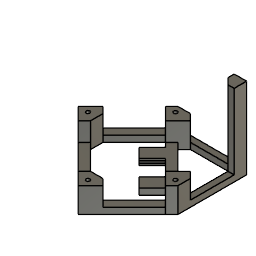
台1 v10 (Autodesk Fusion 360 design; units mm, degrees)
Autodesk Fusion 360 part; units mm, degrees
sketch "スケッチ1" plane through (0, 0, 0) normal (0, 0, 1) x (1, 0, 0)
  line L0 (0, 0) -> (-55, 0)
  line L1 (0, 0) -> (0, -5)
  line L2 (-10, -5) -> (-50, -5)
  line L3 (0, 0) -> (0, -55)
  line L4 (-5, -50) -> (-5, -10)
  line L5 (-5, -10) -> (-10, -5)
  line L6 (-5, -50) -> (-50, -5)
  line L7 (-5, -60) -> (-60, -5)
  line L8 (-60, -5) -> (-55, 0)
  line L9 (0, -55) -> (-5, -60)
  constraint coincident L0.start L1.start
  constraint horizontal L0
  constraint perpendicular L0 L1
  constraint perpendicular L1 L2
  constraint perpendicular L0 L3
  constraint perpendicular L2 L4
  constraint parallel L6 L7
  constraint perpendicular L6 L8
  constraint perpendicular L7 L9
extrude "押し出し1" add sketch "スケッチ1" along normal blind 5
sketch "スケッチ2" plane through (0, 0, 0) normal (0, 0, 1) x (1, 0, 0)
  line L0 (0, 0, 5) -> (-55, 0, 5)
  line L1 (-10, -5, 5) -> (-10, 0, 5)
  line L2 (-10, -5, 5) -> (-5, -10, 5)
  line L3 (0, -55, 5) -> (0, 0, 5)
  line L4 (-5, -10, 5) -> (0, -10, 5)
  line L5 (-60, -5, 5) -> (-5, -60, 5)
  line L6 (-5, -60, 5) -> (0, -55, 5)
  line L7 (-55, 0, 5) -> (-60, -5, 5)
  line L8 (-10, -55, 5) -> (-15, -50, 5)
  line L9 (-5, -10, 5) -> (-5, -50, 5)
  line L10 (0, -45, 5) -> (-5, -40, 5)
  line L11 (-15, -50, 5) -> (-5, -40, 5)
  line L12 (-50, -5, 5) -> (-10, -5, 5)
  line L13 (-50, -15, 5) -> (-40, -5, 5)
  line L14 (-45, 0, 5) -> (-40, -5, 5)
  line L15 (-55, -10, 5) -> (-50, -15, 5)
  point P0 (-10, -5)
  point P1 (-10, -5)
  point P2 (-5, -10)
  point P3 (-5, -50)
  point P4 (-50, -5)
  constraint coincident P0 P1
  constraint coincident P1 P0
extrude "押し出し2" add sketch "スケッチ2" along normal blind 50 contours L0 L1 L2 L3 L4 | L0 L5 L7 L13 L14 L15 | L3 L5 L6 L8 L10 L11 in plane through (0, 0, 5) normal (0, 0, 1)
sketch "スケッチ3" plane through (0, 0, 0) normal (0, 0, 1) x (1, 0, 0)
extrude "押し出し3" cut 2 faces at (-50, -5, 55) (-5, -50, 55) along direction (0, 0, -1) blind 30
sketch "スケッチ4" plane through (0, 0, 0) normal (0, 0, 1) x (1, 0, 0)
  line L0 (-60, -5) -> (-95, -40)
  line L1 (-95, -40) -> (-40, -95)
  line L2 (-40, -95) -> (-5, -60)
  line L3 (-5, -60) -> (-60, -5)
  line L4 (-55, -10) -> (-80, -35)
  line L5 (-80, -45) -> (-45, -80)
  line L6 (-35, -80) -> (-10, -55)
  line L7 (-35, -80) -> (-45, -80)
  line L8 (-80, -35) -> (-80, -45)
  point P0 (-5, -60)
  constraint perpendicular L0 L1
  constraint coincident P0 L2.end
  constraint coincident L3 L4.start
  constraint perpendicular L3 L4
  constraint perpendicular L4 L5
  constraint coincident L3 L6.end
  constraint perpendicular L3 L6
  constraint horizontal L7
  constraint perpendicular L7 L8
extrude "押し出し4" add sketch "スケッチ4" along normal blind 5 contours L0 L1 L2 L3 L4 L5 L6 L7 L8
sketch "スケッチ5" plane through (0, 0, 5) normal (0, 0, 1) x (-1, 0, 0)
  line L0 (55, 10) -> (60, 5)
  line L1 (60, 5) -> (95, 40)
  line L2 (95, 40) -> (40, 95)
  line L3 (40, 95) -> (5, 60)
  line L4 (10, 55) -> (35, 80)
  line L5 (35, 80) -> (45, 80)
  line L6 (45, 80) -> (80, 45)
  line L7 (80, 45) -> (80, 35)
  line L8 (80, 35) -> (55, 10)
  line L9 (80, 35) -> (85, 30)
  line L10 (80, 45) -> (85, 50)
  line L11 (45, 80) -> (50, 85)
  line L12 (35, 80) -> (30, 85)
  line L13 (5, 60) -> (10, 55)
  constraint coincident L7.end L8.start
  constraint coincident L1 L9.end
  constraint perpendicular L1 L9
  constraint coincident L6.end L7.start
  constraint coincident L2 L10.end
  constraint perpendicular L2 L10
  constraint coincident L5.end L6.start
  constraint coincident L2 L11.end
  constraint perpendicular L2 L11
  constraint coincident L4.end L5.start
  constraint coincident L3 L12.end
  constraint perpendicular L3 L12
extrude "押し出し5" add sketch "スケッチ5" along normal blind 20 contours L1 L2 L7 L9 L10 | L2 L3 L5 L11 L12
extrude "押し出し6" cut 4 faces at (-50, -5, 25) (-85, -40, 25) (-40, -85, 25) (-5, -50, 25) along direction (0, 0, -1) blind 5
extrude "押し出し7" add 2 faces at (-6.6667, -45, 5) (-45, -6.6667, 5) along direction (0, 0, -1) blind 5
sketch "スケッチ6" plane through (0, 0, 20) normal (0, 0, 1) x (-1, 0, 0)
  line L0 (45, 80) -> (50, 85)
  line L1 (50, 85) -> (40, 95)
  line L2 (40, 95) -> (30, 85)
  line L3 (30, 85) -> (35, 80)
  line L4 (35, 80) -> (45, 80)
  circle A0 centre (40, 87) radius 1.5
  circle A1 centre (5, 52) radius 1.5
  circle A2 centre (87, 40) radius 1.5
  circle A3 centre (52, 5) radius 1.5
extrude "押し出し8" cut sketch "スケッチ6" against normal blind 10 contours A0 | A1 | A2 | A3
sketch "スケッチ7" plane through (0, 0, 10) normal (0, 0, 1) x (-1, 0, 0)
  circle A0 centre (40, 87) radius 1.5
  circle A1 centre (40, 87) radius 2.5
  circle A2 centre (87, 40) radius 2.5
  circle A3 centre (87, 40) radius 1.5
  circle A4 centre (5, 52) radius 2.5
  circle A5 centre (5, 52) radius 1.5
  circle A6 centre (52, 5) radius 2.5
  circle A7 centre (52, 5) radius 1.5
  constraint concentric A0 A1
  constraint concentric A2 A3
  constraint concentric A4 A5
  constraint concentric A6 A7
extrude "押し出し9" cut sketch "スケッチ7" against normal blind 10 contours A0 | A1 | A2 | A3 | A4 | A5 | A6 | A7
extrude "押し出し10" cut 4 faces at (-38.0024, -87.8241, 10) (-2.8482, -51.8013, 10) (-54.1518, -4.8013, 10) (-85.2875, -41.3179, 10) along direction (0, 0, 1) blind 5
extrude "押し出し11" add 1 faces at (-5, -5, 55) along direction (0, 0, 1) blind 30
sketch "スケッチ8" plane through (-7.5, -7.5, 0) normal (-0.707107, -0.707107, 0) x (0.707107, -0.707107, 0)
  line L0 (-3.5355, 0) -> (3.5355, 0)
  line L1 (3.5355, 0) -> (3.5355, 5)
  line L2 (3.5355, 5) -> (3.5355, 85)
  line L3 (3.5355, 85) -> (-3.5355, 85)
  line L4 (-3.5355, 85) -> (-3.5355, 5)
  line L5 (-3.5355, 5) -> (-3.5355, 0)
  line L6 (0, 35) -> (0, 25)
  line L7 (-1.5, 35) -> (-1.5, 25)
  arc A0 (-1.5, 25) -> (1.5, 25) centre (0, 25) ccw
  line L8 (1.5, 25) -> (1.5, 35)
  arc A1 (1.5, 35) -> (-1.5, 35) centre (0, 35) ccw
  line L9 (0, 35) -> (0, 25) construction
  constraint perpendicular L0 L6
  constraint tangent L7 A0
  constraint tangent A0 L8
  constraint parallel L7 L8
  constraint tangent L8 A1
  constraint tangent L7 A1
  constraint coincident L6.end A0.centre
  constraint parallel L6 L9
  constraint coincident L6.start A1.centre
extrude "押し出し12" cut sketch "スケッチ8" against normal blind 4 contours L7 A0 L8 A1
sketch "スケッチ9" plane through (-32.5, -32.5, 0) normal (-0.707107, -0.707107, 0) x (0.707107, -0.707107, 0)
  line L0 (-24.7487, 20) -> (-38.8909, 20)
  line L1 (-38.8909, 20) -> (-38.8909, 5)
  line L2 (-38.8909, 5) -> (-31.8198, 5)
  line L3 (-31.8198, 5) -> (-31.8198, 0)
  line L4 (-31.8198, 0) -> (31.8198, 0)
  line L5 (31.8198, 0) -> (31.8198, 5)
  line L6 (31.8198, 5) -> (38.8909, 5)
  line L7 (38.8909, 5) -> (38.8909, 20)
  line L8 (38.8909, 20) -> (24.7487, 20)
  line L9 (24.7487, 20) -> (24.7487, 5)
  line L10 (24.7487, 5) -> (-24.7487, 5)
  line L11 (-24.7487, 5) -> (-24.7487, 20)
  line L12 (-9, 5) -> (-20, 5)
  line L13 (-20, 5) -> (-20, 0)
  line L14 (-20, 0) -> (-9, 0)
  line L15 (-9, 0) -> (-9, 5)
  line L16 (9, 5) -> (20, 5)
  line L17 (20, 5) -> (20, 0)
  line L18 (20, 0) -> (9, 0)
  line L19 (9, 0) -> (9, 5)
  constraint horizontal L12
  constraint vertical L13
  constraint horizontal L14
  constraint vertical L15
  constraint coincident L4 L13.end
  constraint coincident L10 L12.start
  constraint horizontal L16
  constraint vertical L17
  constraint horizontal L18
  constraint vertical L19
  constraint coincident L4 L17.end
  constraint coincident L10 L16.start
extrude "押し出し13" add sketch "スケッチ9" along normal blind 20 contours L4 L10 L12 L13 L14 L15 | L4 L10 L16 L17 L18 L19
sketch "スケッチ10" plane through (-46.6421, -46.6421, 0) normal (-0.707107, -0.707107, 0) x (0.707107, -0.707107, 0)
  line L0 (-9, 0) -> (-9, 5)
  line L1 (-9, 5) -> (-20, 5)
  line L2 (-20, 5) -> (-20, 0)
  line L3 (-20, 0) -> (-9, 0)
  line L4 (-9.5, 2.5) -> (9.5, 2.5)
  line L5 (-9.5, 1.5) -> (9.5, 1.5)
  arc A0 (9.5, 1.5) -> (9.5, 3.5) centre (9.5, 2.5) ccw
  line L6 (9.5, 3.5) -> (-9.5, 3.5)
  arc A1 (-9.5, 3.5) -> (-9.5, 1.5) centre (-9.5, 2.5) ccw
  line L7 (-9.5, 2.5) -> (9.5, 2.5) construction
  constraint perpendicular L0 L4
  constraint tangent L5 A0
  constraint tangent A0 L6
  constraint parallel L5 L6
  constraint tangent L6 A1
  constraint tangent L5 A1
  constraint coincident L4.end A0.centre
  constraint perpendicular L0 L7
  constraint coincident L4.start A1.centre
extrude "押し出し14" cut sketch "スケッチ10" against normal blind 20 contours L0 L5 L6 A1 | L0 L5 A0 L6
extrude "押し出し15" cut 2 faces at (-58.5444, -34.7398, 2.5249) (-34.7398, -58.5444, 2.4751) along direction (0.707107, 0.707107, 0) blind 5
sketch "スケッチ11" plane through (0, 0, 0) normal (0, 0, -1) x (1, 0, 0)
  line L0 (-49.4706, 36.7426) -> (-57.2487, 28.9645)
  line L1 (-57.2487, 28.9645) -> (-46.6421, 18.3579)
  line L2 (-46.6421, 18.3579) -> (-55, 10)
  line L3 (-55, 10) -> (-80, 35)
  line L4 (-80, 35) -> (-80, 45)
  line L5 (-80, 45) -> (-45, 80)
  line L6 (-45, 80) -> (-35, 80)
  line L7 (-35, 80) -> (-10, 55)
  line L8 (-10, 55) -> (-18.3579, 46.6421)
  line L9 (-18.3579, 46.6421) -> (-28.9645, 57.2487)
  line L10 (-28.9645, 57.2487) -> (-36.7426, 49.4706)
  line L11 (-36.7426, 49.4706) -> (-26.136, 38.864)
  line L12 (-26.136, 38.864) -> (-38.864, 26.136)
  line L13 (-38.864, 26.136) -> (-49.4706, 36.7426)
  line L14 (-5, 60) -> (-40, 95)
  line L15 (-40, 95) -> (-95, 40)
  line L16 (-95, 40) -> (-55, 0)
  line L17 (-55, 0) -> (0, 0)
  line L18 (0, 0) -> (0, 55)
  line L19 (0, 55) -> (-5, 60)
  line L20 (-5, 10) -> (-10, 5)
  line L21 (-10, 5) -> (-40, 5)
  line L22 (-40, 5) -> (-45, 10)
  line L23 (-45, 10) -> (-10, 45)
  line L24 (-10, 45) -> (-5, 40)
  line L25 (-5, 40) -> (-5, 10)
  circle A0 centre (-40, 87) radius 2.5
  circle A1 centre (-87, 40) radius 2.5
  circle A2 centre (-5, 52) radius 2.5
  circle A3 centre (-52, 5) radius 2.5
extrude "押し出し16" cut 1 faces at (-5, -5, 85) along direction (0, 0, -1) blind 20
sketch "スケッチ12" plane through (0, 0, 0) normal (0, 0, -1) x (1, 0, 0)
  line L0 (-49.4706, 36.7426) -> (-57.2487, 28.9645)
  line L1 (-57.2487, 28.9645) -> (-46.6421, 18.3579)
  line L2 (-46.6421, 18.3579) -> (-55, 10)
  line L3 (-55, 10) -> (-80, 35)
  line L4 (-80, 35) -> (-80, 45)
  line L5 (-80, 45) -> (-45, 80)
  line L6 (-45, 80) -> (-35, 80)
  line L7 (-35, 80) -> (-10, 55)
  line L8 (-10, 55) -> (-18.3579, 46.6421)
  line L9 (-18.3579, 46.6421) -> (-28.9645, 57.2487)
  line L10 (-28.9645, 57.2487) -> (-36.7426, 49.4706)
  line L11 (-36.7426, 49.4706) -> (-26.136, 38.864)
  line L12 (-26.136, 38.864) -> (-38.864, 26.136)
  line L13 (-38.864, 26.136) -> (-49.4706, 36.7426)
  line L14 (-5, 60) -> (-40, 95)
  line L15 (-40, 95) -> (-95, 40)
  line L16 (-95, 40) -> (-55, 0)
  line L17 (-55, 0) -> (0, 0)
  line L18 (0, 0) -> (0, 55)
  line L19 (0, 55) -> (-5, 60)
  line L20 (-5, 10) -> (-10, 5)
  line L21 (-10, 5) -> (-40, 5)
  line L22 (-40, 5) -> (-45, 10)
  line L23 (-45, 10) -> (-10, 45)
  line L24 (-10, 45) -> (-5, 40)
  line L25 (-5, 40) -> (-5, 10)
  circle A0 centre (-40, 87) radius 2.5
  circle A1 centre (-87, 40) radius 2.5
  circle A2 centre (-5, 52) radius 2.5
  circle A3 centre (-52, 5) radius 2.5
  circle A4 centre (-52, 5) radius 3.5
  circle A5 centre (-5, 52) radius 3.5
  circle A6 centre (-40, 87) radius 3.5
  circle A7 centre (-87, 40) radius 3.5
  constraint concentric A3 A4
  constraint concentric A2 A5
  constraint concentric A0 A6
  constraint concentric A1 A7
extrude "押し出し17" cut sketch "スケッチ12" against normal blind 15 contours A4 | A5 | A6 | A7
